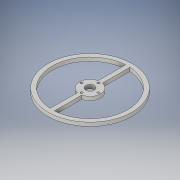
# Autodesk Inventor part: AcrylicFlywheel4
Saved by Autodesk Inventor 2018 (Build 220112000, 112)
## iProperties
Created: 2019-06-24
Part Number: AcrylicFlywheel4
Material: Generic
Document SubType Name: Modeling
Designer: anirudh
Density: 1 g/cm^3
Appearance: Default
Author: anirudh
Autodesk Inventor part; units mm, degrees
ref_plane "YZ Plane" through (0, 0, 0) normal (1, 0, 0) x (0, 1, 0)
ref_plane "XZ Plane" through (0, 0, 0) normal (0, 1, 0) x (-1, 0, 0)
ref_plane "XY Plane" through (0, 0, 0) normal (0, 0, 1) x (1, 0, 0)
sketch "Sketch1" plane through (0, 0, 0) normal (0, 1, 0) x (-1, 0, 0)
  circle A0 centre (0, 0) radius 63.5
  circle A1 centre (0, 0) radius 6.35
  circle A2 centre (-12.7, 0) radius 1.75
  circle A3 centre (0, -12.7) radius 1.75
  circle A4 centre (12.7, 0) radius 1.75
  circle A5 centre (0, 12.7) radius 1.75
  dimension "d8" = 3.5
  dimension "d9" = 3.5
  dimension "d10" = 3.5
  dimension "d11" = 3.5
  constraints: 6 centre point, 2 coincident
  measures "d8" diameter of A2
  measures "d9" diameter of A3
  measures "d10" diameter of A4
  measures "d11" diameter of A5
extrude "Extrusion1" add sketch "Sketch1" along normal blind 5.588
sketch "Sketch2" plane through (0, 5.588, 0) normal (0, 1, 0) x (1, 0, 0)
  arc A0 (-4.7625, 15.1438) -> (-4.7625, -15.1438) centre (0, 0) ccw
  arc A1 (4.7625, -15.1438) -> (4.7625, 15.1438) centre (0, 0) ccw
  arc A2 (-4.7625, 56.9512) -> (-4.7625, -56.9512) centre (0, 0) ccw
  arc A3 (4.7625, -56.9512) -> (4.7625, 56.9512) centre (0, 0) ccw
  arc A4 (3.175, -57.0617) -> (3.175, 57.0617) centre (0, 0) ccw
  arc A5 (-3.175, 57.0617) -> (-3.175, -57.0617) centre (0, 0) ccw
  line L0 (-3.175, 57.0617) -> (-3.175, 15.5543)
  line L1 (-3.175, -15.5543) -> (-3.175, -57.0617)
  line L2 (3.175, 57.0617) -> (3.175, 15.5543)
  line L3 (3.175, -15.5543) -> (3.175, -57.0617)
  arc A6 (-3.175, 15.5543) -> (-3.175, -15.5543) centre (0, 0) ccw
  arc A7 (3.175, -15.5543) -> (3.175, 15.5543) centre (0, 0) ccw
  constraints: 18 point on circle, 8 centre point, 8 end point, 4 coincident
extrude "Extrusion4" cut sketch "Sketch2" against normal blind 25.4
body "Solid1"
